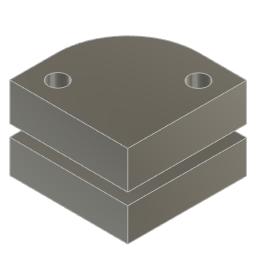
flash glass v1 (Autodesk Fusion 360 design; units mm, degrees)
Autodesk Fusion 360 part; units mm, degrees
sketch "Sketch1" plane through (0, 0, 0) normal (0, 0, 1) x (1, 0, 0)
  line L0 (0, 0) -> (0.1076, 29.9998)
  line L1 (0, 0) -> (-29.9998, 0.1076)
  circle A0 centre (0, 0) radius 30
  line L2 (0.1076, 29.9998) -> (20.1075, 29.9281)
  line L3 (-29.9998, 0.1076) -> (-30.0716, -19.8923)
  line L4 (-30.0716, -19.8923) -> (19.9281, -20.0716)
  line L5 (19.9281, -20.0716) -> (20.1075, 29.9281)
  line L6 (10.1076, 29.9639) -> (9.9282, -20.0357) construction
  line L7 (-30.0357, -9.8923) -> (19.964, -10.0717) construction
  line L8 (10.0968, 26.964) -> (3.8051, 23.3615)
  line L9 (3.8051, 23.3615) -> (3.7791, 16.1115)
  line L10 (3.7791, 16.1115) -> (10.0448, 12.464)
  line L11 (10.0448, 12.464) -> (16.3364, 16.0665)
  line L12 (16.3364, 16.0665) -> (16.3624, 23.3165)
  line L13 (16.3624, 23.3165) -> (10.0968, 26.964)
  line L14 (-23.4332, -16.1947) -> (-16.1833, -16.2207)
  line L15 (-27.0357, -9.9031) -> (-23.4332, -16.1947)
  line L16 (-23.3882, -3.6374) -> (-27.0357, -9.9031)
  line L17 (-16.1382, -3.6634) -> (-23.3882, -3.6374)
  line L18 (-12.5358, -9.9551) -> (-16.1382, -3.6634)
  line L19 (-16.1833, -16.2207) -> (-12.5358, -9.9551)
  circle A1 centre (-19.7857, -9.9291) radius 4.05
  circle A2 centre (10.0708, 19.714) radius 4.05
  point P0 (10.0708, 19.714)
  point P1 (-19.7857, -9.9291)
  dimension "d2" = 30
  dimension "d3" = 30
  dimension "d4" = 20
  dimension "d5" = 20
  dimension "d6" = 7.25
  dimension "d8" = 3
  dimension "d9" = 7.25
  dimension "d10" = 3
  dimension "d11" = 8.1
  dimension "d12" = 8.1
  constraint coincident L0.start L1.start
  constraint perpendicular L0 L1
  constraint coincident L0.end A0
  constraint perpendicular L0 L2
  constraint perpendicular L1 L3
  constraint perpendicular L3 L4
  constraint perpendicular L2 L5
  constraint midpoint L2 L6.start
  constraint coincident L4 L6.end
  constraint perpendicular L4 L6
  constraint midpoint L3 L7.start
  constraint coincident L5 L7.end
  constraint perpendicular L3 L7
  constraint coincident L6 P0
  constraint parallel L6 L9
  constraint parallel L4 L14
  constraint coincident L7 P1
  constraint coincident P1 A1.centre
  constraint coincident P0 A2.centre
  measures "d2" distance of L0.start L0.end
  measures "d3" distance of L0.start L1.end
  measures "d4" distance of L0.end L2.end
  measures "d5" distance of L1.end L3.end
  measures "d6" distance of L8.start P0
  measures "d8" distance of L6.start L8.start
  measures "d9" distance of P1 L17.start
  measures "d10" distance of L3 L15.start
  measures "d11" diameter of A1
  measures "d12" diameter of A2
extrude "Extrude1" add sketch "Sketch1" along normal blind 8 contours L0 L1 A0 L4 L5 | A0 L2 L5 | A0 L3 L4 | L8 L9 L10 L11 L12 L13 | L14 L15 L16 L17 L18 L19 makes body 1
extrude "Extrude2" add sketch "Sketch1" against normal blind 6 contours L0 L1 A0 | L0 L1 A0 L4 L5 | A0 L2 L5 | A0 L3 L4 bodies 1
extrude "Extrude3" add sketch "Sketch1" along normal blind 8 separate body contours L0 L1 A0 | L0 L1 A0 L4 L5 | A0 L2 L5 | A0 L3 L4 | L8 L9 L10 L11 L12 L13 | L14 L15 L16 L17 L18 L19 makes body 2
extrude "Extrude4" add sketch "Sketch1" against normal blind 8 contours L0 L1 A0 L4 L5 | A0 L2 L5 | A0 L3 L4 | L8 L9 L10 L11 L12 L13 | L14 L15 L16 L17 L18 L19 bodies 2
move_body "Move1" bodies 1 to x (1, 0, 0) y (0, 1, 0) z (0, 0, 1) at (0, 0, -21)
sketch "Sketch2" plane through (0, 0, 8) normal (0, 0, 1) x (-1, 0, 0)
  circle A0 centre (-10.0708, -19.714) radius 4.05
  circle A1 centre (19.7857, 9.9291) radius 4.05
  arc A2 (-0.1076, -29.9998) -> (29.9998, -0.1076) centre (0, 0) ccw
  line L0 (29.9998, -0.1076) -> (30.0716, 19.8923)
  line L1 (30.0716, 19.8923) -> (-19.9281, 20.0716)
  line L2 (-19.9281, 20.0716) -> (-20.1075, -29.9281)
  line L3 (-20.1075, -29.9281) -> (-0.1076, -29.9998)
  circle A3 centre (19.7857, 9.9291) radius 4
  circle A4 centre (19.7857, 9.9291) radius 5.6442
  dimension "d24" = 8
  constraint concentric A1 A3
  constraint concentric A1 A4
  measures "d24" diameter of A3
extrude "Extrude5" add sketch "Sketch2" against normal up to surface (35 mm away) separate body contours A3 makes body 3
extrude "Extrude6" add sketch "Sketch2" along normal blind 4 contours A1 | A3 | A4 bodies 3
thread "Thread1" "ISO Metric profile 8.0 M8x1.25 6g" major diameter 7.866 minor diameter 6.4455 pitch 1.25 angle 60 modelled right hand crest width 0.1833 on face at (-23.7659, -9.5308, -15.3333) crest through (-23.7187, -9.9291, 8.3125) on bodies 3
sketch "Sketch3" plane through (0, 0, 12) normal (0, 0, 1) x (-1, 0, 0)
  circle A0 centre (19.7857, 9.9291) radius 5.6442
  circle A1 centre (19.7857, 9.9291) radius 5.6442
  line L0 (17, 7) -> (20.9295, 6.052)
  line L1 (20.9295, 6.052) -> (23.7153, 8.9811)
  line L2 (23.7153, 8.9811) -> (22.5715, 12.8582)
  line L3 (22.5715, 12.8582) -> (18.642, 13.8062)
  line L4 (18.642, 13.8062) -> (15.8562, 10.8771)
  line L5 (15.8562, 10.8771) -> (17, 7)
  point P0 (19.7857, 9.9291)
  constraint coincident P0 A0.centre
extrude "Extrude7" cut sketch "Sketch3" against normal blind 3 contours L0 L1 L2 L3 L4 L5 bodies 3
hidden bodies 3
equation "d6 = ( 14.5 / 2 ) * 1 mm"
equation "d9 = ( 14.5 / 2 ) * 1 mm"
named bodies: "top", "bottom"
